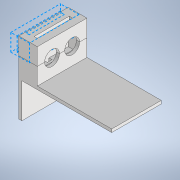
# Autodesk Inventor part: snapConnector
Saved by Autodesk Inventor 2022 (Build 260153000, 153)
## iProperties
Created: 2022-06-03
Part Number: snapConnector
Material: Generic
Document SubType Name: Modeling
Designer: tecware
Density: 1 g/cm^3
Appearance: Default
Author: tecware
## iProperties of the stored document snapConnector_3DPrint.ipt
Created: 2022-06-03
Part Number: snapConnector_3DPrint
Material: Generic
Document SubType Name: Modeling
Designer: tecware
Density: 1 g/cm^3
Appearance: Default
Author: tecware
Autodesk Inventor part; units mm, degrees
ref_plane "YZ Plane" through (0, 0, 0) normal (1, 0, 0) x (0, 1, 0)
ref_plane "XZ Plane" through (0, 0, 0) normal (0, 1, 0) x (-1, 0, 0)
ref_plane "XY Plane" through (0, 0, 0) normal (0, 0, 1) x (1, 0, 0)
sketch "Sketch2" plane through (0, 0, 0) normal (1, 0, 0) x (0, 1, 0)
  line L0 (11, -16) -> (-11, -16)
  line L1 (-11, -16) -> (-11, 16)
  line L2 (-11, 16) -> (11, 16)
  line L3 (11, 16) -> (11, -16)
  line L4 (11, -16) -> (-11, 16) construction
  line L5 (-11, -16) -> (11, 16) construction
  circle A0 centre (0, -6.5) radius 4.8
  circle A1 centre (0, 6.5) radius 4.8
  line L6 (0, 6.5) -> (0, 0)
  point P0 (0, 0)
  dimension "d8" = 22
  dimension "d9" = 32
  dimension "d14" = 9.6
  dimension "d15" = 13
  dimension "d23" = 6.5
  dimension "d24" = 9.6
  dimension "d25" = 13
  constraints: 14 end point, 2 centre point, 2 midpoint, 2 perpendicular, 1 coincident
  measures "d8" distance of L1.end L2.end
  measures "d9" distance of L0.end L1.end
  measures "d14" diameter of A1
  measures "d15" distance of point (0, -6.5) L6.start
  measures "d23" distance of L6.start L6.end
  measures "d24" diameter of A0
  measures "d25" distance of A0.centre L6.start
extrude "Extrusion2" add sketch "Sketch2" against normal blind 10
shell "Shell1" thickness 2 removed faces 3 at (-10, 8.8868, -1.7838) at (-6.6667, 4.7378, -7.27) at (-6.6667, 4.7378, 5.73)
sketch "Sketch4" plane through (0, 0, 0) normal (0, 1, 0) x (-1, 0, 0)
  line L0 (2, -14) -> (2, 14) projected
  line L1 (2, 0) -> (4.75, 0) construction
  line L2 (4.75, -11.3497) -> (6.75, -11.3497)
  line L3 (6.75, -11.3497) -> (6.75, 11.3497)
  line L4 (6.75, 11.3497) -> (4.75, 11.3497)
  line L5 (4.75, 11.3497) -> (4.75, -11.3497)
  point P0 (0, 0)
  dimension "d19" = 2.75
  dimension "d20" = 2
  constraints: 10 end point, 2 midpoint
  measures "d19" distance of L1.start L1.end
  measures "d20" distance of L4.end L3.end
extrude "Extrusion4" [suppressed]
sketch "Sketch5" plane through (0, -11, -16) normal (0, -1, 0) x (1, 0, 0)
  line L0 (-10, 2) -> (-10, 30) projected
  line L1 (-8, 17.5) -> (-10, 17.5)
  line L2 (-10, 17.5) -> (-10, 14.5)
  line L3 (-10, 14.5) -> (-8, 14.5)
  line L4 (-8, 14.5) -> (-8, 17.5)
  line L5 (-8, 17.5) -> (-10, 14.5) construction
  line L6 (-10, 17.5) -> (-8, 14.5) construction
  line L7 (-10, 0) -> (-10, 32) projected
  point P0 (0, 16)
  dimension "d27" = 3
  dimension "d30" = 2
  constraints: 12 end point, 2 perpendicular, 1 collinear, 1 point on line
  measures "d27" distance of L2.end L1.end
  measures "d30" distance of L2.end L3.end
extrude "Extrusion5" cut sketch "Sketch5" against normal blind 2
sketch "Sketch6" plane through (-2, -9, 14) normal (-1, 0, 0) x (0, 0, 1)
  line L0 (0, 18) -> (0, 0) projected
  line L1 (-28, 16) -> (0, 16)
  line L2 (0, 16) -> (0, 2)
  line L3 (0, 2) -> (-28, 2)
  line L4 (-28, 2) -> (-28, 16)
  line L5 (-28, 16) -> (0, 2) construction
  line L6 (0, 16) -> (-28, 2) construction
  line L7 (-28, 18) -> (0, 18)
  line L8 (0, 18) -> (0, 0)
  line L9 (0, 0) -> (-28, 0)
  line L10 (-28, 0) -> (-28, 18)
  line L11 (-28, 18) -> (0, 0) construction
  line L12 (0, 18) -> (-28, 0) construction
  point P0 (-14, 9)
  dimension "d31" = 14
  constraints: 24 end point, 4 midpoint, 1 point on line
  measures "d31" distance of L1.end L2.end
extrude "Extrusion6" add sketch "Sketch6" along normal blind 2.75 contours L0 L1 L10 L7 | L0 L9 L10 L3
sketch "Sketch7" plane through (0, -11, -16) normal (0, -1, 0) x (1, 0, 0)
  circle A0 centre (37, 7.4) radius 2.5 projected
  circle A1 centre (3, 24.6) radius 2.5 projected
  line L0 (-10, 14.5) -> (-10, 0) projected
  line L1 (-10, 0) -> (48, 0) projected
  line L2 (48, 0) -> (48, 32) projected
  line L3 (48, 32) -> (-10, 32) projected
  line L4 (-10, 32) -> (-10, 17.5) projected
  line L5 (-10, 17.5) -> (-8, 17.5) projected
  line L6 (-8, 17.5) -> (-8, 14.5) projected
  line L7 (-8, 14.5) -> (-10, 14.5) projected
  line L8 (-6.75, 4.6503) -> (-6.75, 27.3497) projected
  line L9 (-6.75, 27.3497) -> (-4.75, 27.3497) projected
  line L10 (-4.75, 27.3497) -> (-4.75, 4.6503) projected
  line L11 (-4.75, 4.6503) -> (-6.75, 4.6503) projected
  line L12 (-10, 0) -> (-10, 32) projected
  point P0 (0, 16)
extrude "Extrusion7" add sketch "Sketch7" along normal blind 2 contours A0 | A1 | L7 L6 L5 L4 L3 L2 L1 L0 | L8 L9 L10 L11
sketch "Sketch8" plane through (-10, 0, 0) normal (-1, 0, 0) x (0, 0, 1)
  line L0 (16, 11) -> (-16, 11) projected
  line L1 (-16, 11) -> (-16, -35.4) projected
  line L2 (16, -35.4) -> (-16, -35.4) projected
  line L3 (16, 11) -> (16, -35.4) projected
  point P0 (0, 0)
extrude "Extrusion8" add sketch "Sketch8" along normal blind 2
sketch "Sketch9" plane through (0, -13, -16) normal (0, -1, 0) x (1, 0, 0)
  circle A0 centre (37, 7.4) radius 1.4 projected
  circle A1 centre (37, 7.4) radius 2.5 projected
  circle A2 centre (3, 24.6) radius 1.4 projected
  circle A3 centre (3, 24.6) radius 2.5 projected
  point P0 (0, 16)
extrude "Extrusion9" add sketch "Sketch9" along normal blind 4
sketch "Sketch10" plane through (0, 0, 0) normal (1, 0, 0) x (0, 0, -1)
  line L0 (-16, 11) -> (-16, -11) projected
  line L1 (-16, -11) -> (16, -11) projected
  line L2 (16, -11) -> (16, 11) projected
  line L3 (16, 11) -> (-16, 11) projected
  circle A0 centre (-6.5, 0) radius 4.8 projected
  circle A1 centre (6.5, 0) radius 4.8 projected
  line L4 (16, -11) -> (16, 11) projected
  line L5 (16, 0) -> (-16, 0)
  line L6 (-16, -35.4) -> (-16, 11) projected
  line L7 (-16, 11) -> (16, 11)
  line L8 (16, 11) -> (16, 0)
  line L9 (16, 0) -> (-16, 0)
  line L10 (-16, 0) -> (-16, 11)
  point P0 (0, 0)
  point P1 (11.3, 0)
  point P2 (-11.3, 0)
  point P3 (-1.7, 0)
  point P4 (1.7, 0)
  constraints: 10 end point, 1 midpoint, 1 point on line
extrude "Extrusion10" cut sketch "Sketch10" against normal blind 12 contours L3 L2 L5 A1 A0 L0 | A0 L5 | L5 A1 picked at (-5.9326, 1.496) picked at (7.6976, 1.061)
sketch "Sketch11" plane through (-8, -9, 1.5) normal (0, 1, 0) x (1, 0, 0)
  line L0 (1.45, 12.6493) -> (1.45, -9.6497) projected
  line L1 (3.05, 12.6493) -> (1.45, 12.6493) projected
  line L2 (1.45, -9.6497) -> (3.05, -9.6497) projected
  line L3 (1.45, 12.6493) -> (3.2385, 12.6493)
  line L4 (3.2385, 12.6493) -> (3.2385, -9.6497)
  line L5 (3.2385, -9.6497) -> (1.45, -9.6497)
  line L6 (1.45, -9.6497) -> (1.45, 12.6493)
  point P0 (8, 1.5)
  constraints: 8 end point, 1 point on line
extrude "Extrusion11" [suppressed]
sketch "Sketch12" plane through (0, 0, -11.3) normal (0, 1, 0) x (1, 0, 0)
  line L0 (-2, -9.6) -> (0, -9.6) projected
  line L1 (-2, -13) -> (-2, -9.6) projected
  line L2 (0, -13) -> (-2, -13) projected
  line L3 (0, -9.6) -> (0, -13) projected
  line L4 (0, 0) -> (-2, 0) projected
  line L5 (0, 4.7) -> (0, 0) projected
  line L6 (-12, 4.7) -> (0, 4.7) projected
  line L7 (-12, -27.3) -> (-12, 4.7) projected
  line L8 (0, -27.3) -> (-12, -27.3) projected
  line L9 (0, -22.6) -> (0, -27.3) projected
  line L10 (-2, -22.6) -> (0, -22.6) projected
  line L11 (-2, -25.3) -> (-2, -22.6) projected
  line L12 (-10, -25.3) -> (-2, -25.3) projected
  line L13 (-10, 2.7) -> (-10, -25.3) projected
  line L14 (-2, 2.7) -> (-10, 2.7) projected
  line L15 (-2, 0) -> (-2, 2.7) projected
  point P0 (0, -11.3)
extrude "Extrusion12" add sketch "Sketch12" along normal blind 11
body "Solid1"
